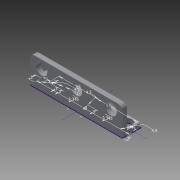
# Autodesk Inventor part: Bar
Saved by Autodesk Inventor 2014 SP1 (Build 180222100, 222)
## iProperties
Created: 2015-03-26
Part Number: Bar
Material: Generic
Document SubType Name: Modeling
Designer: Erin
Density: 1 g/cm^3
Appearance: Default
Author: Erin
Autodesk Inventor part; units mm, degrees
ref_plane "YZ Plane" through (0, 0, 0) normal (1, 0, 0) x (0, 1, 0)
ref_plane "XZ Plane" through (0, 0, 0) normal (0, 1, 0) x (-1, 0, 0)
ref_plane "XY Plane" through (0, 0, 0) normal (0, 0, 1) x (1, 0, 0)
sketch "Sketch1" plane through (0, 0, 0) normal (0, 0, 1) x (1, 0, 0)
  line L0 (-20, -3) -> (20, -3) construction
  circle A0 centre (-17, 0) radius 2.25
  circle A1 centre (17, 0) radius 2.25
  circle A2 centre (0, 0) radius 2.25
  circle A3 centre (-7, 0.3446) radius 1
  circle A4 centre (7, 0.3446) radius 1
  line L1 (-23.9554, 0) -> (25.6733, 0) construction
  line L2 (0, 11.421) -> (0, -11.2937) construction
  line L3 (-20, -3) -> (20, -3)
  line L4 (20, -3) -> (20, 3)
  line L5 (20, 3) -> (-20, 3)
  line L6 (-20, 3) -> (-20, -3)
  circle A5 centre (-11.8345, 1.6861) radius 0.5
  line L7 (-20, -3) -> (20, -3)
  line L8 (20, -3) -> (20, -5)
  line L9 (20, -5) -> (-20, -5)
  line L10 (-20, -5) -> (-20, -3)
  point P0 (0, 0)
  point P1 (0, -3)
  point P2 (0, -3)
  point P3 (-2.8751, -5.808)
  point P4 (2.8751, -5.808)
  dimension "d0" = 40
  dimension "d1" = 4.5
  dimension "d2" = 4.5
  dimension "d3" = 3
  dimension "d4" = 4.5
  dimension "d5" = 3
  dimension "d6" = 3.3446
  dimension "d7" = 3.3446
  dimension "d8" = 3
  dimension "d9" = 17
  dimension "d10" = 17
  dimension "d11" = 3
  dimension "d12" = 3
  dimension "d13" = 3
  dimension "d14" = 3
  dimension "d16" = 1
  dimension "d20" = 2
  constraints: 22 end point, 6 centre point, 5 parallel, 3 horizontal, 3 perpendicular, 2 point on line, 1 coincident, 1 collinear, 1 midpoint, 1 vertical
  measures "d0" distance of L0.start L0.end
  measures "d1" diameter of A0
  measures "d2" diameter of A1
  measures "d3" distance from line of A0.centre L0
  measures "d4" diameter of A2
  measures "d5" distance from line of A2.centre L0
  measures "d6" distance from line of A3.centre L0
  measures "d7" distance from line of A4.centre L0
  measures "d8" distance between parallel lines of L0 L1
  measures "d9" distance from line of L2 A1.centre
  measures "d10" distance from line of L2 A0.centre
  measures "d11" distance from line of A0.centre L3
  measures "d12" distance from line of A0.centre L6
  measures "d13" distance from line of A0.centre L5
  measures "d14" distance from line of A1.centre L4
  measures "d16" diameter of A5
  measures "d20" distance of L7.end L8.end
extrude "Extrusion1" add sketch "Sketch1" along normal blind 2 contours L6 L5 L4 L3
extrude "Extrusion2" add sketch "Sketch1" along normal blind 12 contours L3 L8 L9 L10
sketch "Sketch2" plane through (-20, -3, 2) normal (0, 1, 0) x (1, 0, 0)
  line L0 (0, 0) -> (40, 0) projected
  line L1 (0, 0) -> (0, -10)
  line L2 (40, -10) -> (0, -10) projected
  line L3 (40, 0) -> (40, -10)
  circle A0 centre (5, -6.5) radius 2.5
  circle A1 centre (35, -6.5) radius 2.5
  line L4 (20, 0) -> (20, -10) construction
  line L5 (0, -6.5) -> (40, -6.5) construction
  circle A2 centre (20, -6.5) radius 2.5
  point P0 (20, 2)
  dimension "d24" = 5
  dimension "d25" = 5
  dimension "d26" = 15
  dimension "d27" = 15
  dimension "d28" = 3.5
  dimension "d29" = 5
  constraints: 8 end point, 4 point on line, 3 centre point, 3 midpoint, 1 perpendicular
  measures "d24" diameter of A0
  measures "d25" diameter of A1
  measures "d26" distance from line of L4 A0.centre
  measures "d27" distance from line of A1.centre L4
  measures "d28" distance between parallel lines of L2 L5
  measures "d29" diameter of A2
extrude "Extrusion3" cut sketch "Sketch2" against normal blind 7 contours A0 | A1 | A2
fillet "Fillet2" radius 2 2 edges at (20, -4, 12) (-20, -4, 12)
fillet "Fillet3" radius 1 2 edges at (20, 3, 1) (-20, 3, 1)
body "Solid1"
